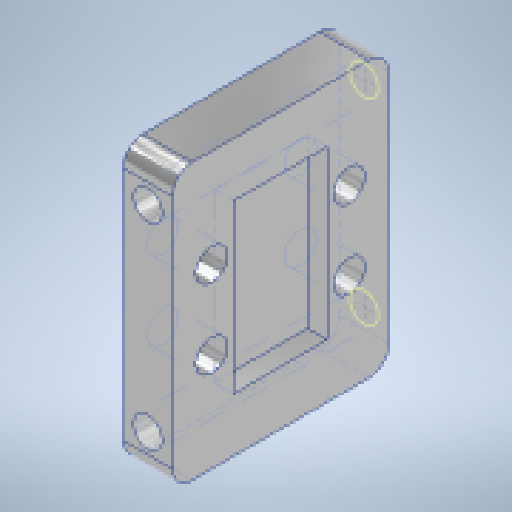
# Autodesk Inventor part: belt_holder_1
Saved by Autodesk Inventor 2025 (Build 290162000, 162)
## iProperties
Created: 2025-02-25
Part Number: belt_holder_1
Material: アルミニウム 6061
Document SubType Name: Modeling
Designer: Zhopa
Density: 2.7 g/cm^3
Appearance: アルミニウム - フラット
Mass: 6.1235 g
Surface Area: 23.371 cm^2
Volume: 2.26796 cm^3
Author: Zhopa
Autodesk Inventor part; units mm, degrees
ref_plane "YZ Plane" through (0, 0, 0) normal (1, 0, 0) x (0, 1, 0)
ref_plane "XZ Plane" through (0, 0, 0) normal (0, 1, 0) x (-1, 0, 0)
ref_plane "XY Plane" through (0, 0, 0) normal (0, 0, 1) x (1, 0, 0)
sketch "Sketch1" plane through (0, 0, 0) normal (1, 0, 0) x (0, 1, 0)
  line L0 (0, 0) -> (28, 0)
  line L1 (28, 0) -> (28, -22)
  line L2 (28, -22) -> (0, -22)
  line L3 (0, -22) -> (0, 0)
  dimension "d0" = 28
  dimension "d1" = 22
  constraints: 8 end point, 2 parallel, 1 horizontal, 1 perpendicular
  measures "d0" distance of L1.end L2.end
  measures "d1" distance of L0.end L1.end
extrude "Extrusion1" add sketch "Sketch1" along normal blind 5
sketch "Sketch2" plane through (0, 0, 0) normal (0, 0, 1) x (1, 0, 0)
  line L0 (0, 28) -> (5, 28) projected
  line L1 (0, 0) -> (5, 0) projected
  point P0 (2.5, 4)
  point P1 (2.5, 24)
  dimension "d4" = 4
  dimension "d5" = 4
  measures "d4" distance from line of point (2.5, 24) L0
  measures "d5" distance from line of L1 point (2.5, 4)
hole "Hole1" at (2.5, 4, 0) at (2.5, 24, 0) direction (0, 0, -1) diameter 3 depth 80.45
sketch "Sketch3" plane through (5, 0, 0) normal (1, 0, 0) x (0, 0, -1)
  line L0 (22, 28) -> (0, 28) projected
  line L1 (0, 0) -> (22, 0) projected
  line L2 (0, 28) -> (0, 0) projected
  line L3 (11, 28) -> (11, 0)
  point P0 (4, 18)
  point P1 (4, 10)
  point P2 (18, 18)
  point P3 (18, 10)
  dimension "d13" = 10
  dimension "d14" = 10
  dimension "d15" = 4
  dimension "d16" = 4
  constraints: 2 end point, 2 midpoint, 2 symmetric about line
  measures "d13" distance from line of point (4, 18) L0
  measures "d14" distance from line of point (4, 10) L1
  measures "d15" distance from line of point (4, 18) L2
  measures "d16" distance from line of L2 point (4, 10)
hole "Hole2" at (5, 18, -4) at (5, 10, -4) at (5, 18, -18) at (5, 10, -18) direction (-1, 0, 0) diameter 3.2 depth 80.45
fillet "Fillet1" radius 2 4 edges at (2.5, 28, 0) (2.5, 28, -22) (2.5, 0, -22) (2.5, 0, 0)
sketch "Sketch4" plane through (5, 0, 0) normal (1, 0, 0) x (0, 0, -1)
  circle A0 centre (4, 18) radius 1.6 projected
  circle A1 centre (18, 10) radius 1.6 projected
  line L0 (4, 18) -> (18, 18)
  line L1 (18, 18) -> (18, 10)
  line L2 (18, 10) -> (4, 10)
  line L3 (4, 10) -> (4, 18)
  line L4 (22, 22.5) -> (0, 22.5) projected
  line L5 (15.75, 5.5) -> (6.25, 5.5)
  line L6 (6.25, 5.5) -> (6.25, 22.5)
  line L7 (6.25, 22.5) -> (15.75, 22.5)
  line L8 (15.75, 22.5) -> (15.75, 5.5)
  line L9 (15.75, 5.5) -> (6.25, 22.5) construction
  line L10 (6.25, 5.5) -> (15.75, 22.5) construction
  line L11 (6.25, 22.5) -> (15.75, 22.5)
  line L12 (15.75, 22.5) -> (15.75, 29.5007)
  line L13 (15.75, 29.5007) -> (6.25, 29.5007)
  line L14 (6.25, 29.5007) -> (6.25, 22.5)
  line L15 (6.25, 5.5) -> (15.75, 5.5)
  line L16 (15.75, 5.5) -> (15.75, -2.0044)
  line L17 (15.75, -2.0044) -> (6.25, -2.0044)
  line L18 (6.25, -2.0044) -> (6.25, 5.5)
  point P0 (0, 0)
  point P1 (11, 14)
  dimension "d25" = 9.5
  constraints: 36 end point, 8 parallel, 4 horizontal, 4 perpendicular, 2 midpoint, 2 point on line
  measures "d25" distance of L6.end L7.end
extrude "Extrusion2" cut sketch "Sketch4" against normal blind 2 contours L6 L4 L8 L0 | L0 L8 L2 L6 | L2 L8 L5 L6
sketch "Sketch5" plane through (0, 2, -22) normal (0, 0, -1) x (-1, 0, 0)
  circle A0 centre (-2.5, 2) radius 1.5 projected
  circle A1 centre (-2.5, 22) radius 1.5 projected
  point P0 (0, -2)
  constraints: 2 coincident
body "Solid1"
